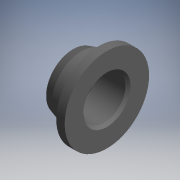
# Autodesk Inventor part: 80F-0503
Saved by Autodesk Inventor 2017.3 (Build 213256000, 256)
## iProperties
Part Number: 80F-0503
Material: Generic
Catalog Web Link: www.cadenas.de
Description: Flange Bushings-80F
Vendor: OILES
Document SubType Name: Modeling
Designer: partserver
Manufacturer: OILES
Mass: 0.110779 g
Surface Area: 2.66414 cm^2
Volume: 0.110779 cm^3
Density: 1 g/cm^3
Appearance: PSOLRGB-127-127-127
Category: PARTsolutions
Company: OILES
Title: 80F-0503
Author: Cadenas PARTsolutions
Comments: 80F
PSOL_IDENT_0: {$CADENAS_DATA\23d-libs\oiles\plastic_bearings\oiles_80\flange_bushings_80b.prj},166 {VTYP=3D},{NB=8
PSOL_IDENT_1: 0F-0503},{LINA=80F-0503},{NN=Flange Bushings},{DATE=15.04.2019 22:54:28},{GEOMDATE=07.11.2016 06:24:
PSOL_IDENT_2: 13},{VERSION=},{LINEID=120},{WBVAR=},{WBNUMERIC=}  {NB=80F-0503},{LINA=80F-0503},{KT=DUMMY},{ORDERNO=
PSOL_IDENT_3: 80F-0503},{S=5},{SRT=h7(0/-0.012)},{H=7},{HRT=H7(+0.015/0)},{ID=5},{IDT=+0.095/+0.045},{OD=7},{ODT=+
PSOL_IDENT_4: 0.157/+0.045},{F=10},{FT=1.0},{FTT=0/-0.10},{L=3},{LT=0/-0.3},{A=0.3},{B=1.0},{C=C0.3},{CC=0.300},{C
PSOL_IDENT_5: R=0.000},{TE=-40~80°C},{P=17.5N/mm2  (179kgf/cm2)},{V=0.85m/s  (51m/min)},{PV=2.45N/mm2•m/s  (1,500k
PSOL_IDENT_6: gf/cm2•m/min)},{AIT=The inner diameter tolerances are the values after pressing into a ring gauge of
PSOL_IDENT_7: OD+-0.002},{CAU=Please refer to catalog about detail.}
NB: 80F-0503
NN: Flange Bushings
NT: 80F
NBSYN: $ORDERNO.
LINA: 80F-0503
CATALOG: OILES CORPORATION
ORDERNO: 80F-0503
S: 5
SRT: h7(0/-0.012)
H: 7
HRT: H7(+0.015/0)
ID: 5
IDT: +0.095/+0.045
OD: 7
ODT: +0.157/+0.045
F: 10
FT: 1
FTT: 0/-0.10
L: 3
LT: 0/-0.3
TE: -40~80°C
P: 17.5N/mm2  (179kgf/cm2)
V: 0.85m/s  (51m/min)
PV: 2.45N/mm2•m/s  (1,500kgf/cm2•m/min)
AIT: The inner diameter tolerances are the values after pressing into a ring gauge of OD+-0.002.
CAU: Please refer to catalog about detail.
SUPPLIER: OILES
ARTICLENO: 80F-0503
BOMINFO: 80F-0503
CREATOR: CADENAS GmbH
Autodesk Inventor part; units mm, degrees
ref_plane "YZ Plane" through (0, 0, 0) normal (1, 0, 0) x (0, 1, 0)
ref_plane "XZ Plane" through (0, 0, 0) normal (0, 1, 0) x (-1, 0, 0)
ref_plane "XY Plane" through (0, 0, 0) normal (0, 0, 1) x (1, 0, 0)
sketch "Sketch_1" plane through (0, 0, 0) normal (0, 0, 1) x (1, 0, 0)
  line L0 (4, 0) -> (0, 0)
  line L1 (0, 2.8) -> (0.3, 2.5)
  line L2 (0.3, 2.5) -> (3.7, 2.5)
  line L3 (3.7, 2.5) -> (4, 2.8)
  line L4 (4, 2.8) -> (4, 3.2)
  line L5 (4, 3.2) -> (3, 3.5)
  line L6 (3, 3.5) -> (1, 3.5)
  line L7 (1, 3.5) -> (1, 5)
  line L8 (1, 5) -> (0, 5)
  line L9 (0, 5) -> (0, 2.8)
  constraints: 20 end point
revolve "Revolution1" add sketch "Sketch_1" angle 360 about axis through (4, 0, 0) along (1, 0, 0)
body "Solid1"
